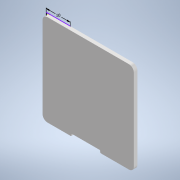
# Autodesk Inventor part: ButerBoard
Saved by Autodesk Inventor 2022 (Build 260153000, 153)
## iProperties
Created: 2024-07-26
Part Number: ButerBoard
Material: Типовые
Document SubType Name: Modeling
Designer: Капустяник Андрей
Density: 1 g/cm^3
Appearance: По умолчанию
Author: Капустяник Андрей
Autodesk Inventor part; units mm, degrees
ref_plane "YZ Plane" through (0, 0, 0) normal (1, 0, 0) x (0, 1, 0)
ref_plane "XZ Plane" through (0, 0, 0) normal (0, 1, 0) x (-1, 0, 0)
ref_plane "РабПлоскость1" through (0, 0, 3.5) normal (0, 0, 1) x (1, 0, 0)
sketch "Эскиз1" plane through (0, 0, 3.5) normal (0, 0, 1) x (1, 0, 0)
  line L0 (-19, -19) -> (19, -19)
  line L1 (19, -19) -> (19, 19)
  line L2 (19, 19) -> (-19, 19)
  line L3 (-19, 19) -> (-19, -19)
  line L4 (-19, -19) -> (19, 19) construction
  line L5 (19, -19) -> (-19, 19) construction
  point P0 (0, 0)
  dimension "d1" = 38
  dimension "d2" = 38
  constraints: 12 end point, 2 midpoint, 2 parallel, 1 horizontal, 1 perpendicular
  measures "d1" distance of L2.end L1.end
  measures "d2" distance of L1.end L0.end
extrude "Выдавливание1" add sketch "Эскиз1" along normal blind 1.5
fillet "Сопряжение1" radius 2 4 edges at (19, -19, 4.25) (19, 19, 4.25) (-19, 19, 4.25) (-19, -19, 4.25)
sketch "Эскиз2" plane through (0, 0, 3.5) normal (0, 0, -1) x (-1, 0, 0)
  line L0 (19, 17) -> (19, -17) projected
  line L1 (19, 0) -> (13, 0)
  line L2 (-17, 19) -> (17, 19) projected
  line L3 (13, 19) -> (13, -19)
  line L4 (17, -19) -> (-17, -19) projected
  line L5 (7, -19) -> (-5, -19)
  line L6 (-19, -19) -> (1, -19)
  line L7 (-19, -17) -> (-19, 17) projected
  line L8 (7, -20) -> (-5, -20)
  line L9 (-5, -20) -> (-5, -18)
  line L10 (-5, -18) -> (7, -18)
  line L11 (7, -18) -> (7, -20)
  line L12 (7, -20) -> (-5, -18) construction
  line L13 (-5, -20) -> (7, -18) construction
  point P0 (0, 0)
  point P1 (-5, -19)
  dimension "d6" = 6
  dimension "d7" = 12
  dimension "d8" = 20
  dimension "d9" = 2
  constraints: 20 end point, 6 midpoint, 4 point on line, 3 horizontal, 2 parallel, 1 collinear, 1 perpendicular, 1 vertical
  measures "d6" distance of L1.start L1.end
  measures "d7" distance of L5.start L5.end
  measures "d8" distance of L6.end L6.start
  measures "d9" distance of L8.end L9.end
extrude "Выдавливание2" cut sketch "Эскиз2" against normal blind 1.5 contours L4 L9 L10 L11
fillet "Сопряжение2" radius 0.3 4 edges at (-7, -19, 4.25) (-7, -18, 4.25) (5, -19, 4.25) (5, -18, 4.25)
sketch "Эскиз3" plane through (0, 0, 3.5) normal (0, 0, -1) x (-1, 0, 0)
  arc A0 (19, 17) -> (17, 19) centre (17, 17) ccw projected
  line L0 (19, 17) -> (19, 19)
  line L1 (19, 19) -> (9, 19)
  line L2 (9, 19) -> (9, -19)
  line L3 (17, -19) -> (7.3, -19) projected
  point P0 (0, 0)
  dimension "d13" = 10
  constraints: 6 end point, 2 perpendicular, 1 point on line, 1 tangent, 1 vertical
  measures "d13" distance of L0.end L1.end
